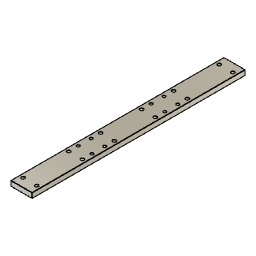
Spacer bar (Autodesk Fusion 360 design; units mm, degrees)
Autodesk Fusion 360 part; units mm, degrees
sketch "Top" plane through (0, 0, 0) normal (0, 0, 1) x (1, 0, 0)
  line L0 (0, 0) -> (25, 0)
  line L1 (25, 0) -> (25, 500)
  line L2 (25, 500) -> (-25, 500)
  line L3 (-25, 500) -> (-25, 0)
  line L4 (-25, 0) -> (0, 0)
  line L5 (-16, 0) -> (-16, 500) construction
  line L6 (16, 0) -> (16, 500) construction
  line L7 (0, 0) -> (0, 500) construction
  line L8 (0, 20) -> (16, 20) construction
  line L9 (0, 20) -> (-16, 20) construction
  line L10 (-16, 127) -> (16, 127) construction
  line L11 (16, 149.5) -> (-16, 149.5) construction
  line L12 (-16, 179.5) -> (16, 179.5) construction
  line L13 (-16, 202) -> (16, 202) construction
  line L14 (-16, 298) -> (16, 298) construction
  line L15 (-16, 320.5) -> (16, 320.5) construction
  line L16 (-16, 350.5) -> (16, 350.5) construction
  line L17 (-16, 373) -> (16, 373) construction
  line L18 (-16, 480) -> (16, 480) construction
  circle A0 centre (-16, 149.5) radius 3
  circle A1 centre (-16, 179.5) radius 3
  circle A2 centre (16, 149.5) radius 3
  circle A3 centre (16, 179.5) radius 3
  circle A4 centre (-16, 320.5) radius 3
  circle A5 centre (16, 320.5) radius 3
  circle A6 centre (-16, 350.5) radius 3
  circle A7 centre (16, 350.5) radius 3
  circle A8 centre (-16, 480) radius 3.5
  circle A9 centre (16, 480) radius 3.5
  circle A10 centre (-16, 373) radius 3.5
  circle A11 centre (16, 373) radius 3.5
  circle A12 centre (-16, 298) radius 3.5
  circle A13 centre (16, 298) radius 3.5
  circle A14 centre (-16, 202) radius 3.5
  circle A15 centre (16, 202) radius 3.5
  circle A16 centre (-16, 127) radius 3.5
  circle A17 centre (16, 127) radius 3.5
  circle A18 centre (-16, 20) radius 3.5
  circle A19 centre (16, 20) radius 3.5
  dimension "d1" = 50
  dimension "d2" = 500
  dimension "d3" = 32
  dimension "d4" = 20
  dimension "d5" = 107
  dimension "d6" = 22.5
  dimension "d7" = 22.5
  dimension "d8" = 30
  dimension "d9" = 22.5
  dimension "d10" = 22.5
  dimension "d11" = 30
  dimension "d12" = 107
  dimension "d13" = 20
  dimension "d14" = 96
  dimension "d15" = 6
  dimension "d16" = 6
  dimension "d18" = 6
  dimension "d19" = 6
  dimension "d20" = 6
  dimension "d21" = 6
  dimension "d22" = 6
  dimension "d23" = 6
  dimension "d24" = 7
  dimension "d25" = 7
  dimension "d26" = 7
  dimension "d27" = 7
  dimension "d28" = 7
  dimension "d29" = 7
  dimension "d30" = 7
  dimension "d31" = 7
  dimension "d32" = 7
  dimension "d33" = 7
  dimension "d34" = 7
  dimension "d35" = 7
  constraint coincident L0.start L4.end
  constraint horizontal L0
  constraint perpendicular L0 L1
  constraint perpendicular L1 L2
  constraint perpendicular L2 L3
  constraint perpendicular L3 L4
  constraint equal L0 L4
  constraint coincident L4 L5.start
  constraint coincident L2 L5.end
  constraint perpendicular L2 L5
  constraint coincident L0 L6.start
  constraint coincident L2 L6.end
  constraint perpendicular L2 L6
  constraint midpoint L2 L7.end
  constraint coincident L7 L8.start
  constraint coincident L6 L8.end
  constraint perpendicular L6 L8
  constraint coincident L5 L9.end
  constraint perpendicular L5 L9
  constraint equal L8 L9
  constraint coincident L5 L10.start
  constraint coincident L6 L10.end
  constraint perpendicular L6 L10
  constraint coincident L6 L11.start
  constraint coincident L5 L11.end
  constraint perpendicular L5 L11
  constraint coincident L5 L12.start
  constraint coincident L6 L12.end
  constraint perpendicular L6 L12
  constraint coincident L5 L13.start
  constraint coincident L6 L13.end
  constraint perpendicular L6 L13
  constraint coincident L5 L14.start
  constraint coincident L6 L14.end
  constraint perpendicular L6 L14
  constraint coincident L5 L15.start
  constraint coincident L6 L15.end
  constraint perpendicular L6 L15
  constraint coincident L5 L16.start
  constraint coincident L6 L16.end
  constraint perpendicular L6 L16
  constraint coincident L5 L17.start
  constraint coincident L6 L17.end
  constraint perpendicular L6 L17
  constraint coincident L5 L18.start
  constraint coincident L6 L18.end
  constraint perpendicular L6 L18
  constraint coincident L11.end A0.centre
  constraint coincident L12.start A1.centre
  constraint coincident L11.start A2.centre
  constraint coincident L12.end A3.centre
  constraint coincident L15.start A4.centre
  constraint coincident L15.end A5.centre
  constraint coincident L16.start A6.centre
  constraint coincident L16.end A7.centre
  constraint coincident L18.start A8.centre
  constraint coincident L18.end A9.centre
  constraint coincident L17.start A10.centre
  constraint coincident L17.end A11.centre
  constraint coincident L14.start A12.centre
  constraint coincident L14.end A13.centre
  constraint coincident L13.start A14.centre
  constraint coincident L13.end A15.centre
  constraint coincident L10.start A16.centre
  constraint coincident L10.end A17.centre
  constraint coincident L9.end A18.centre
  constraint coincident L8.end A19.centre
  measures "d1" distance of L1.end L2.end
  measures "d2" distance of L2.end L3.end
  measures "d3" distance of L5 L6
  measures "d4" distance of L4 L9
  measures "d5" distance of L9 L10
  measures "d6" distance of L10 L11
  measures "d7" distance of L12 L13
  measures "d8" distance of L11 L12
  measures "d9" distance of L16 L17
  measures "d10" distance of L14 L15
  measures "d11" distance of L15 L16
  measures "d12" distance of L17 L18
  measures "d13" distance of L2 L18
  measures "d14" distance of L13 L14
  measures "d15" diameter of A0
  measures "d16" diameter of A1
  measures "d18" diameter of A2
  measures "d19" diameter of A3
  measures "d20" diameter of A4
  measures "d21" diameter of A5
  measures "d22" diameter of A6
  measures "d23" diameter of A7
  measures "d24" diameter of A8
  measures "d25" diameter of A9
  measures "d26" diameter of A10
  measures "d27" diameter of A11
  measures "d28" diameter of A12
  measures "d29" diameter of A13
  measures "d30" diameter of A14
  measures "d31" diameter of A15
  measures "d32" diameter of A16
  measures "d33" diameter of A17
  measures "d34" diameter of A18
  measures "d35" diameter of A19
extrude "Extrude1" add sketch "Top" along normal blind 12
chamfer "Chamfer1" distance 0.5 angle 45 12 edges at (0, 0, 12) (25, 250, 12) (-25, 250, 12) (25, 0, 6) (-25, 0, 6) (0, 0, 0) (25, 250, 0) (25, 500, 6) (0, 500, 12) (0, 500, 0) (-25, 500, 6) (-25, 250, 0)
chamfer "Chamfer2" distance 0.5 angle 45 20 edges at (-19.2631, 21.2657, 12) (12.7369, 21.2657, 12) (-19.2631, 128.2657, 12) (-18.797, 150.5848, 12) (-18.797, 180.5848, 12) (-19.2631, 203.2657, 12) (12.7369, 128.2657, 12) (13.203, 150.5848, 12) (13.203, 180.5848, 12) (12.7369, 203.2657, 12) (-19.2631, 299.2657, 12) (-18.797, 321.5848, 12) (-18.797, 351.5848, 12) (-19.2631, 374.2657, 12) (12.7369, 299.2657, 12) (13.203, 321.5848, 12) (13.203, 351.5848, 12) (12.7369, 374.2657, 12) (12.7369, 481.2657, 12) (-19.2631, 481.2657, 12)
chamfer "Chamfer3" distance 0.5 angle 45 20 edges at (12.7369, 21.2657, 0) (-19.2631, 21.2657, 0) (12.7369, 128.2657, 0) (-19.2631, 128.2657, 0) (-18.797, 150.5848, 0) (-18.797, 180.5848, 0) (-19.2631, 203.2657, 0) (13.203, 150.5848, 0) (13.203, 180.5848, 0) (12.7369, 203.2657, 0) (12.7369, 299.2657, 0) (13.203, 321.5848, 0) (13.203, 351.5848, 0) (12.7369, 374.2657, 0) (-19.2631, 299.2657, 0) (-18.797, 321.5848, 0) (-18.797, 351.5848, 0) (-19.2631, 374.2657, 0) (-19.2631, 481.2657, 0) (12.7369, 481.2657, 0)
named bodies: "Plate"
